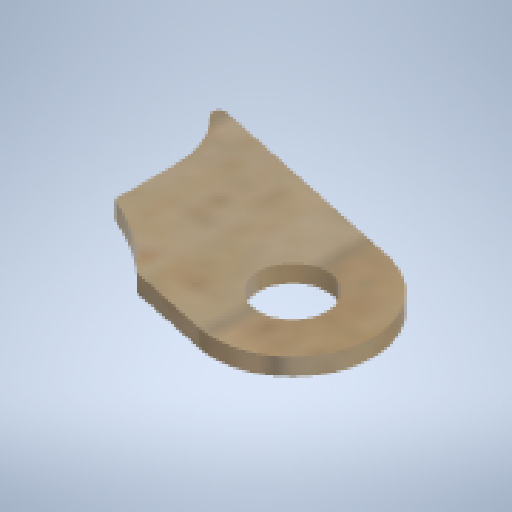
# Autodesk Inventor part: gear_plate_3
Saved by Autodesk Inventor 2026.1 (Build 301233020, 233B)
## iProperties
Created: 2024-04-01
Part Number: gear_plate_3
Material: 木材 (カエデ材)
Document SubType Name: Modeling
Designer: hibik
Density: 0.67 g/cm^3
Appearance: ナチュラル カエデ材 - 光沢 濃い着色
Author: hibik
Autodesk Inventor part; units mm, degrees
ref_plane "YZ Plane" through (0, 0, 0) normal (1, 0, 0) x (0, 1, 0)
ref_plane "XZ Plane" through (0, 0, 0) normal (0, 1, 0) x (-1, 0, 0)
ref_plane "XY Plane" through (0, 0, 0) normal (0, 0, 1) x (1, 0, 0)
sketch "スケッチ1" plane through (0, 0, 0) normal (0, 1, 0) x (-1, 0, 0)
  line L0 (25, 0) -> (-25, 0)
  line L1 (-25, 0) -> (-25, -104.5)
  line L2 (-25, -104.5) -> (25, -104.5)
  line L3 (25, -104.5) -> (25, 0)
  circle A0 centre (0, 0) radius 25
  circle A1 centre (0, 0) radius 57 construction
  circle A2 centre (0, 0) radius 75 construction
  circle A3 centre (0, 0) radius 10.75
  circle A4 centre (-77.746127, -62.893082) radius 25
  circle A5 centre (-77.746127, -62.893082) radius 10.75
  line L4 (-77.746127, -62.893082) -> (-82.968428, -87.341549)
  line L5 (-82.968428, -87.341549) -> (-5.222301, -103.948468)
  line L6 (5.222301, -55.051532) -> (-72.523826, -38.444614)
  circle A6 centre (0, -79.5) radius 25
  circle A7 centre (0, 0) radius 82
  circle A8 centre (0, 0) radius 65
  line L7 (-48.165066, -43.647753) -> (-96.972293, -33.222313)
  line L8 (-96.972293, -33.222313) -> (-92.794452, -13.663539)
  line L9 (-92.794452, -13.663539) -> (-43.987225, -24.088979)
  line L10 (-43.987225, -24.088979) -> (-48.165066, -43.647753)
  line L11 (-96.972293, -33.222313) -> (-102.194595, -57.67078)
  point P0 (-25, -79.5)
  point P1 (-25, -48.595915)
  point P2 (-25, -60)
  point P3 (-48.165066, -43.647753)
  point P4 (-61.75052, -20.294661)
  dimension "d22" = 130
  dimension "d0" = 114
  dimension "d2" = 150
  dimension "d4" = 21.5
  dimension "d5" = 50
  dimension "d19" = 79.5
  dimension "d20" = 79.5
  dimension "d21" = 164
  dimension "d23" = 20
  constraints: 24 end point, 10 tangent, 8 centre point, 8 coincident, 6 point on circle, 4 parallel, 3 perpendicular, 2 equal radius, 2 point on line, 1 collinear, 1 horizontal, 1 midpoint, 3 other
  measures "d0" diameter of A1
  measures "d2" diameter of A2
  measures "d4" diameter of A3
  measures "d5" distance of L1.end L2.end
  measures "d19" distance of point (0, 0) A6.centre
  measures "d20" distance from line of A6.centre L4
  measures "d21" diameter of A7
  measures "d23" distance between parallel lines of L7 L9
sketch "スケッチ1 outline for 押し出し1" plane through (0, 0, 0) normal (0, 1, 0) x (-1, 0, 0)
  arc A0 (-72.523826, -38.444614) -> (-82.968428, -87.341549) centre (-77.746127, -62.893082) ccw
  line L0 (-82.968428, -87.341549) -> (-5.222301, -103.948468)
  arc A1 (-5.222301, -103.948468) -> (-25, -79.5) centre (0, -79.5) cw
  line L1 (-25, -79.5) -> (-25, -60)
  arc A2 (-25, -60) -> (-48.165066, -43.647753) centre (0, 0) cw
  line L2 (-48.165066, -43.647753) -> (-72.523826, -38.444614)
  circle A3 centre (-77.746127, -62.893082) radius 10.75
extrude "押し出し1" add sketch "スケッチ1 outline for 押し出し1" along normal blind 5.5
fillet "フィレット1" radius 2 1 edges at (5.2223, 2.75, -103.9485)
equation "\"d20\" = d19"
